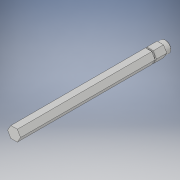
# Autodesk Inventor part: Gearbox_hex_shaft
Saved by Autodesk Inventor 2018 (Build 220112000, 112)
## iProperties
Created: 2018-09-06
Part Number: Gearbox_hex_shaft
Material: Generic
Document SubType Name: Modeling
Designer: baoan
Density: 1 g/cm^3
Appearance: Default
Author: baoan
Autodesk Inventor part; units mm, degrees
ref_plane "YZ Plane" through (0, 0, 0) normal (1, 0, 0) x (0, 1, 0)
ref_plane "XZ Plane" through (0, 0, 0) normal (0, 1, 0) x (-1, 0, 0)
sketch "Sketch1" plane through (0, 0, 0) normal (0, 0, 1) x (1, 0, 0)
  line L0 (-3.6662, 6.35) -> (3.6662, 6.35)
  line L1 (3.6662, 6.35) -> (7.3323, 0)
  line L2 (7.3323, 0) -> (3.6662, -6.35)
  line L3 (3.6662, -6.35) -> (-3.6662, -6.35)
  line L4 (-3.6662, -6.35) -> (-7.3323, 0)
  line L5 (-7.3323, 0) -> (-3.6662, 6.35)
  point P0 (0, 0)
  point P1 (0, 0)
  dimension "d0" = 7.3323
  constraints: 12 end point, 1 coincident, 1 horizontal, 13 other
  measures "d0" distance of L0.start L0.end
extrude "Extrusion1" add sketch "Sketch1" along normal mid plane 166.1414
sketch "Sketch2" plane through (0, 0, -83.0707) normal (0, 0, -1) x (-1, 0, 0)
  circle A0 centre (0, 0) radius 3.175
  circle A1 centre (0, 0) radius 6.35
  dimension "d3" = 6.35
  dimension "d4" = 12.7
  constraints: 2 centre point, 2 coincident
  measures "d3" diameter of A0
  measures "d4" diameter of A1
extrude "Extrusion2" add sketch "Sketch2" along normal blind 6.35
chamfer "Chamfer1" distance 0.7874 angle 45 1 edges at (6.35, 0, -89.4207)
ref_plane "Work Plane1" through (-1.8331, 3.175, 83.0707) normal (0.866, 0.5, 0) x (0, 0, -1)
sketch "Sketch3" plane through (-1.8331, 3.175, 83.0707) normal (0.866, 0.5, 0) x (0, 0, -1)
  line L0 (166.1414, -3.6662) -> (166.1414, 0) projected
  line L1 (154.432, 1.9218) -> (154.432, 5.7318)
  line L2 (152.8445, 1.9218) -> (152.8445, 5.7318)
  line L3 (154.432, 1.9218) -> (159.062, 1.9218) construction
  line L4 (166.1414, -3.6662) -> (163.6991, -3.6662)
  line L5 (154.432, 5.7318) -> (152.8445, 5.7318)
  line L6 (154.432, 1.9218) -> (152.8445, 1.9218)
  point P0 (83.0707, -3.6662)
  dimension "d10" = 11.7094
  dimension "d11" = 1.5875
  dimension "d12" = 5.588
  dimension "d13" = 3.81
  constraints: 12 end point, 3 horizontal, 2 horizontal alignment, 2 vertical, 1 perpendicular
  measures "d10" distance between parallel lines of L1 L0
  measures "d11" distance between parallel lines of L1 L2
  measures "d12" distance between parallel lines of L4 L3
  measures "d13" distance of L2.start L2.end
revolve "Revolution1" cut sketch "Sketch3" angle 360 about axis through (0, 0, -83.0707) along (0, 0, 1)
body "Solid1"
